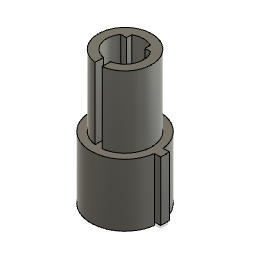
Yamaha AM802 Pot Knob (Autodesk Fusion 360 design; units mm, degrees)
Autodesk Fusion 360 part; units mm, degrees
sketch "Sketch1" plane through (0, 0, 0) normal (0, 1, 0) x (1, 0, 0)
  circle A0 centre (0, 0) radius 5.75
  circle A1 centre (0, 0) radius 4.5
  circle A2 centre (0, 0) radius 3.1
  line L0 (-0.6, -3.0414) -> (-0.6, -4.4598)
  line L1 (0, 0) -> (0, -5.75) construction
  line L2 (0.6, -3.0414) -> (0.6, -4.4598)
  line L3 (0, 0) -> (0, 5.75) construction
  line L4 (0, 3.1) -> (0, 1.8)
  line L5 (0, 1.8) -> (-2.5239, 1.8)
  line L6 (0, 1.8) -> (2.5239, 1.8)
  line L7 (-1.55, 2.6847) -> (-1.55, 1.8)
  line L8 (1.55, 2.6847) -> (1.55, 1.8)
  line L9 (0, 0) -> (5.75, 0) construction
  line L10 (4.75, -0.75) -> (6.75, -0.75)
  line L11 (4.75, 0.75) -> (6.75, 0.75)
  line L12 (4.75, -0.75) -> (4.75, 0.75)
  line L13 (6.75, 0.75) -> (6.75, -0.75)
  dimension "d1" = 11.5
  dimension "d2" = 9
  dimension "d3" = -1.4
  dimension "d5" = 0.6
  dimension "d6" = 1.3
  dimension "d7" = 1.55
  dimension "d15" = 1
  dimension "d17" = 1.5
  dimension "d18" = 2
  constraint coincident A0.centre A1.centre
  constraint concentric A0 A1
  constraint coincident A2 L0.start
  constraint coincident A1 L0.end
  constraint vertical L0
  constraint coincident A0 L1.end
  constraint vertical L1
  constraint symmetric L0.start L1 L2.start
  constraint symmetric L0.end L1 L2.end
  constraint coincident A0 L3.end
  constraint parallel L1 L3
  constraint coincident A2 L4.start
  constraint coincident L3 L4.start
  constraint coincident L3 L4.end
  constraint coincident A2 L5.end
  constraint perpendicular L4 L5
  constraint symmetric L5.start L4 L6.start
  constraint symmetric L4 L5.end L6.end
  constraint coincident A2 L7.start
  constraint coincident L5 L7.end
  constraint perpendicular L5 L7
  constraint symmetric L3 L7.start L8.start
  constraint symmetric L3 L7.end L8.end
  constraint coincident A0 L9.end
  constraint perpendicular L3 L9
  constraint symmetric L9 L10.start L11.start
  constraint symmetric L9 L10.end L11.end
  constraint horizontal L10
  measures "d1" diameter of A0
  measures "d2" diameter of A1
  measures "d5" distance of L0 L1
  measures "d6" distance of L4.start L4.end
  measures "d7" distance of L4 L7
  measures "d15" horizontal distance of L9.end L10.end
  measures "d17" distance of L10.start L11.start
  measures "d18" distance of L10.start L10.end
extrude "Extrude2" add sketch "Sketch1" along normal blind 10 contours A0 L10 L11 L12 | A0 L10 L11 L13 | A0 L10 L11 L12 | A1 A2 L0 L2 | A1 A2 L0 L2 | A2 L5 L6 | A2 L5 L7 | A2 L4 L5 L7 | A2 L6 L8 | A2 L4 L6 L8 makes body 1
extrude "Extrude4" add sketch "Sketch1" against normal blind 0.5 contours A0 L10 L11 L12 | A1 A2 L0 L2 | A1 A2 L0 L2 | A2 L5 L6 | A2 L5 L7 | A2 L4 L5 L7 | A2 L6 L8 | A2 L4 L6 L8 picked at (0.2379, -5.3177) bodies 1
extrude "Extrude1" add sketch "Sketch1" along normal up to surface (22 mm away) separate body contours A1 A2 L0 L2 | A2 L5 L7 | A2 L6 L8 picked at (3.7529, 1.4551) makes body 2
copy_body "Body->Comp1" bodies 2 removing the originals makes body 3 in component "Component"
copy_body "Body->Comp2" bodies 1 removing the originals makes body 4 in component "Knob"
combine "Combine1" operation add target body 4 tool bodies 3 in component "Knob"
component "Knob" placed x (1, 0, 0) y (0, 1, 0) z (0, 0, 1) at (0, 0, 0)
